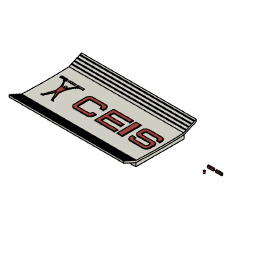
Pen_holder_ceis v9 (Autodesk Fusion 360 design; units mm, degrees)
Autodesk Fusion 360 part; units mm, degrees
sketch "Schizzo3" plane through (0, 0, 0) normal (0, 0, 1) x (1, 0, 0)
  line L0 (0, 0) -> (190, 0)
  line L1 (190, 0) -> (190, 80)
  line L2 (190, 80) -> (0, 80)
  line L3 (0, 80) -> (0, 0)
  dimension "d7" = 80
  dimension "d8" = 190
  constraint horizontal L0
  constraint vertical L1
  constraint horizontal L2
  constraint vertical L3
  constraint coincident L0.start L3.end
  measures "d7" distance of L0.start L2.end
  measures "d8" distance of L1.end L2.end
extrude "Estrusione2" add sketch "Schizzo3" along normal blind 6 makes body 1
sketch "Schizzo4" plane through (190, 0, 0) normal (1, 0, 0) x (0, 1, 0)
  line L0 (0, 0) -> (80, 0)
  line L1 (80, 0) -> (80, 6)
  line L2 (80, 6) -> (0, 6)
  line L3 (0, 6) -> (0, 0)
  line L4 (0, 6) -> (0, 5)
  line L5 (40, 5) -> (40, 9)
  line L6 (-6.5555, 6.3549) -> (30, 25)
  line L7 (30, 25) -> (86.5555, 6.3549)
  arc A0 (-6.5555, 6.3549) -> (86.5555, 6.3549) centre (40, 805.5001) ccw
  constraint coincident L2.end L3.start
  constraint coincident L3 L4.end
  constraint perpendicular L2 L4
  constraint perpendicular L2 L5
  constraint coincident L5.start A0
  constraint coincident L1.end A0
  constraint coincident L2.end A0
extrude "Estrusione3" cut sketch "Schizzo4" against normal through all contours L2 L5 A0 | L2 L6 L7 A0 | L2 L5 A0 bodies 1
sketch "Schizzo5" plane through (190, 0, 0) normal (1, 0, 0) x (0, 1, 0)
  line L0 (80, 0) -> (80, 6)
  line L1 (0, 0) -> (-20, 0)
  line L2 (-20, 0) -> (-20, 15)
  line L3 (80, 0) -> (100, 0)
  line L4 (100, 0) -> (100, 15)
  line L5 (-20, 15) -> (0, 6)
  line L6 (100, 15) -> (80, 6)
  spline S0 degree 5 poles (0, 6) (1.6, 5.9242) (4.8, 5.7791) (9.6, 5.5813) (16, 5.3581) (24, 5.1509) (32, 5.0221) (40, 4.978) (48, 5.0221) (56, 5.1509) (64, 5.3581) (70.4, 5.5813) (75.2, 5.7791) (78.4, 5.9242) (80, 6) knots 0 0 0 0 0 0 0.1 0.2 0.3 0.4 0.5 0.6 0.7 0.8 0.9 1 1 1 1 1 1
  line L7 (-20, 15) -> (-20, 18.2898)
  line L8 (100, 15) -> (100, 18.2898)
  line L9 (-18.7689, 17.7358) -> (0.7109, 8.9698)
  spline S1 degree 3 poles (0.7109, 8.9698) (18.3427, 8.1444) (35.9568, 7.8068) (53.5771, 8.1239) (62.1442, 8.2781) (70.7163, 8.5685) (79.2891, 8.9698) knots 0.007133 0.007133 0.007133 0.007133 0.670389 0.670389 0.670389 0.992867 0.992867 0.992867 0.992867
  line L10 (98.7689, 17.7358) -> (79.2891, 8.9698)
  line L11 (98.7689, 17.7358) -> (100, 18.2898)
  line L12 (-18.7689, 17.7358) -> (-20, 18.2898)
  line L13 (0.7109, 8.9698) -> (-2.9367, 10.6113)
  line L14 (-2.9367, 10.6113) -> (-2.7316, 11.0673)
  line L15 (-2.7316, 11.0673) -> (-3.6435, 11.4776)
  line L16 (-3.6435, 11.4776) -> (-3.8487, 11.0217)
  line L17 (-3.8487, 11.0217) -> (-7.4964, 12.6631)
  line L18 (-7.4964, 12.6631) -> (-7.2912, 13.1191)
  line L19 (-7.2912, 13.1191) -> (-8.2031, 13.5294)
  line L20 (-8.2031, 13.5294) -> (-8.4083, 13.0735)
  line L21 (-8.4083, 13.0735) -> (-12.056, 14.7149)
  line L22 (-12.056, 14.7149) -> (-11.8508, 15.1709)
  line L23 (-11.8508, 15.1709) -> (-12.7627, 15.5813)
  line L24 (-12.7627, 15.5813) -> (-12.9679, 15.1253)
  line L25 (-12.9679, 15.1253) -> (-16.6156, 16.7668)
  line L26 (-16.6156, 16.7668) -> (-16.4104, 17.2227)
  line L27 (-16.4104, 17.2227) -> (-17.3223, 17.6331)
  line L28 (-17.3223, 17.6331) -> (-17.5275, 17.1771)
  line L29 (0, 0) -> (40, 0)
  line L30 (40, 0) -> (40, -6)
  line L31 (82.9368, 10.6113) -> (82.7316, 11.0673)
  line L32 (82.7316, 11.0673) -> (83.6435, 11.4776)
  line L33 (83.6435, 11.4776) -> (83.8487, 11.0217)
  line L34 (87.2912, 13.1191) -> (88.2031, 13.5294)
  line L35 (87.4964, 12.6631) -> (87.2912, 13.1191)
  line L36 (88.2031, 13.5294) -> (88.4083, 13.0735)
  line L37 (92.056, 14.7149) -> (91.8508, 15.1709)
  line L38 (91.8508, 15.1709) -> (92.7627, 15.5813)
  line L39 (92.7627, 15.5813) -> (92.9679, 15.1253)
  line L40 (96.6156, 16.7668) -> (96.4104, 17.2227)
  line L41 (96.4104, 17.2227) -> (97.3223, 17.6331)
  line L42 (97.3223, 17.6331) -> (97.5275, 17.1771)
  point P0 (40, 5)
  dimension "d18" = 20
  dimension "d19" = 15
  dimension "d20" = 20
  dimension "d22" = 15
  dimension "d37" = 3
  dimension "d38" = 4
  dimension "d39" = 0.5
  dimension "d40" = 1
  dimension "d41" = 0.5
  dimension "d42" = 4
  dimension "d43" = 0.5
  dimension "d44" = 1
  dimension "d45" = 0.5
  dimension "d46" = 4
  dimension "d47" = 0.5
  dimension "d48" = 1
  dimension "d49" = 0.5
  dimension "d50" = 4
  dimension "d51" = 0.5
  dimension "d52" = 1
  dimension "d53" = 0.5
  constraint coincident L1.start L29.start
  constraint horizontal L1
  constraint perpendicular L1 L2
  constraint coincident L0.start L3.start
  constraint perpendicular L0 L3
  constraint perpendicular L3 L4
  constraint coincident L0.end L6.end
  constraint parallel L2 L7
  constraint parallel L4 L8
  constraint parallel L10 L11
  constraint parallel L9 L12
  constraint parallel L9 L13
  constraint perpendicular L9 L14
  constraint perpendicular L14 L15
  constraint perpendicular L15 L16
  constraint perpendicular L16 L17
  constraint perpendicular L17 L18
  constraint perpendicular L18 L19
  constraint perpendicular L19 L20
  constraint perpendicular L20 L21
  constraint perpendicular L9 L22
  constraint perpendicular L22 L23
  constraint perpendicular L23 L24
  constraint perpendicular L24 L25
  constraint perpendicular L9 L26
  constraint perpendicular L26 L27
  constraint perpendicular L27 L28
  constraint parallel L1 L29
  constraint perpendicular L29 L30
  constraint symmetric L13.end L30 L31.start
  constraint symmetric L14.end L30 L31.end
  constraint symmetric L15.end L30 L32.end
  constraint symmetric L16.end L30 L33.end
  constraint symmetric L17.end L30 L35.start
  constraint symmetric L18.end L30 L34.start
  constraint symmetric L19.end L30 L34.end
  constraint symmetric L20.end L30 L36.end
  constraint symmetric L21.end L30 L37.start
  constraint symmetric L22.end L30 L37.end
  constraint symmetric L23.end L30 L38.end
  constraint symmetric L24.end L30 L39.end
  constraint symmetric L25.end L30 L40.start
  constraint symmetric L26.end L30 L40.end
  constraint symmetric L27.end L30 L41.end
  constraint symmetric L28.end L30 L42.end
  measures "d18" distance of L1.start L1.end
  measures "d19" distance of L1.end L2.end
  measures "d20" distance of L0.start L3.end
  measures "d22" distance of L3.end L4.end
  measures "d38" distance of L9.end L13.end
  measures "d39" distance of L13.end L14.end
  measures "d40" distance of L14.end L15.end
  measures "d41" distance of L15.end L16.end
  measures "d42" distance of L16.end L17.end
  measures "d43" distance of L17.end L18.end
  measures "d44" distance of L18.end L19.end
  measures "d45" distance of L19.end L20.end
  measures "d46" distance of L20.end L21.end
  measures "d47" distance of L21.end L22.end
  measures "d48" distance of L22.end L23.end
  measures "d49" distance of L23.end L24.end
  measures "d50" distance of L24.end L25.end
  measures "d51" distance of L25.end L26.end
  measures "d52" distance of L26.end L27.end
  measures "d53" distance of L27.end L28.end
extrude "Estrusione5" add sketch "Schizzo5" against normal blind 190 separate body contours L5 L6 S0 L7 L8 L9 S1 L10 L11 L12 L13 L17 L21 L25 | L10 L40 L41 L42 | L9 L26 L27 L28 | L10 L37 L38 L39 | L9 L22 L23 L24 | L10 L34 L35 L36 | L9 L18 L19 L20 | L10 L31 L32 L33 | L9 L14 L15 L16 makes body 2
ref_plane "Piano di lavoro1" through (0, 0, 10) normal (0, 0, 1) x (1, 0, 0)
sketch "Schizzo8" plane through (0, 0, 10) normal (0, 0, 1) x (1, 0, 0)
  arc A0 (63.5, 56) -> (57.5, 50) centre (63.5, 50) ccw
  arc A1 (84.5, 48.2) -> (82.7, 50) centre (82.7, 48.2) ccw
  arc A2 (63.5, 32) -> (65.3, 30.2) centre (65.3, 32) ccw
  arc A3 (84.5, 24.2) -> (90.5, 30.2) centre (84.5, 30.2) ccw
  line L0 (63.5, 24.2) -> (84.5, 24.2)
  line L1 (63.5, 30.2) -> (65.3, 30.2)
  arc A4 (65.3, 50) -> (63.5, 48.2) centre (65.3, 48.2) ccw
  line L2 (57.5, 50) -> (90.5, 50)
  line L3 (57.5, 50) -> (57.5, 30.2)
  line L4 (57.5, 30.2) -> (90.5, 30.2)
  line L5 (84.5, 56) -> (63.5, 56)
  arc A5 (90.5, 50) -> (84.5, 56) centre (84.5, 50) ccw
  arc A6 (82.7, 30.2) -> (84.5, 32) centre (82.7, 32) ccw
  arc A7 (57.5, 30.2) -> (63.5, 24.2) centre (63.5, 30.2) ccw
  line L6 (84.5, 32) -> (82.7, 32)
  line L7 (84.5, 45.8) -> (90.5, 45.8)
  line L8 (63.5, 56) -> (63.5, 24.2)
  line L9 (84.5, 34.4) -> (90.5, 34.4)
  line L10 (103.5, 24.2) -> (103.5, 56)
  line L11 (97.5, 50) -> (130.5006, 50)
  line L12 (97.5, 43.1) -> (127.823, 43.1)
  line L13 (97.5, 40.1) -> (127.823, 40.1)
  line L14 (97.5, 37.1) -> (127.823, 37.1)
  line L15 (97.5, 24.2) -> (97.5, 56)
  line L16 (97.5, 24.2) -> (97.5, 49.1)
  line L17 (97.5, 56) -> (97.5, 40.1)
  line L18 (97.5, 30.2) -> (130.5, 30.2)
  line L19 (97.5, 24.2) -> (130.5, 24.2)
  line L20 (130.5, 24.2) -> (97.5, 24.2)
  line L21 (127.823, 37.1) -> (127.823, 43.1)
  line L22 (97.5, 56) -> (130.5, 56)
  line L23 (134.5, 41.008) -> (134.5, 24.2)
  line L24 (134.5, 39.175) -> (134.5, 55.9829)
  line L25 (143.5, 24.2) -> (143.5, 40.0915)
  line L26 (143.5, 40.0915) -> (143.5, 55.9829)
  arc A8 (177.5, 35.3) -> (175.7, 37.1) centre (175.7, 35.3) ccw
  line L27 (156.5, 37.1) -> (177.5, 37.1)
  line L28 (177.5, 43.1) -> (156.5, 43.1)
  line L29 (150.5, 50) -> (183.5, 50)
  arc A9 (156.5, 55.9397) -> (150.5603, 50) centre (156.5, 50) ccw
  line L30 (177.5, 56) -> (155.5, 56)
  arc A10 (183.5, 49.999) -> (177.5, 56) centre (177.5, 50) ccw
  arc A11 (183.5, 37.0982) -> (177.5, 43.1) centre (177.5, 37.1) ccw
  arc A12 (177.5, 48.2) -> (175.7, 50) centre (175.7, 48.2) ccw
  line L31 (177.5, 46.4) -> (183.5, 46.4)
  arc A13 (156.5, 44.9) -> (158.3, 43.1) centre (158.3, 44.9) ccw
  arc A14 (150.5, 43.1015) -> (156.5, 37.1) centre (156.5, 43.1) ccw
  line L32 (150.5, 30.2) -> (183.5, 30.2)
  line L33 (155.5, 24.2) -> (177.5, 24.2)
  arc A15 (150.5, 30.2) -> (156.5, 24.2) centre (156.5, 30.2) ccw
  arc A16 (156.5, 32) -> (158.3, 30.2) centre (158.3, 32) ccw
  line L34 (150.5, 33.8) -> (156.5, 33.8)
  arc A17 (177.5, 24.2) -> (183.5, 30.201) centre (177.5, 30.2) ccw
  line L35 (134.5, 55.9829) -> (143.5, 55.9829)
  line L36 (134.5, 24.2) -> (143.5, 24.2)
  line L37 (130.5, 56) -> (130.5006, 50)
  line L38 (130.5, 30.2) -> (130.5, 24.2)
  line L39 (84.5, 56) -> (84.5, 45.8)
  line L40 (84.5, 34.4) -> (84.5, 24.2)
  line L41 (90.5, 30.2) -> (90.5, 34.4)
  line L42 (90.5, 45.8) -> (90.5, 50)
  line L43 (150.5, 50) -> (150.5, 43.0985)
  line L44 (150.5, 33.8) -> (150.5, 30.2)
  line L45 (156.5, 56) -> (156.5, 37.1)
  line L46 (156.5, 33.8) -> (156.5, 24.2)
  line L47 (177.5, 24.2) -> (177.5, 43.1)
  line L48 (177.5, 46.4) -> (177.5, 56)
  line L49 (183.5, 30.199) -> (183.5, 37.1018)
  line L50 (183.5, 46.4) -> (183.5, 50.001)
  line L51 (6.5, 60.5) -> (17.5, 60.5)
  line L52 (17.5, 60.5) -> (17.5, 57.5)
  line L53 (17.5, 57.5) -> (6.5, 57.5)
  line L54 (6.5, 57.5) -> (6.5, 60.5)
  circle A18 centre (25.5, 48) radius 2
  line L55 (25.5, 48) -> (25.5, 66.722)
  line L56 (20, 57.5) -> (25.5, 57.5)
  line L57 (25.5, 57.5) -> (25.5, 60.5)
  line L58 (25.5, 60.5) -> (20, 60.5)
  line L59 (20, 60.5) -> (20, 57.5)
  line L60 (3, 16.5) -> (25.5, 16.5)
  line L61 (25.5, 16.5) -> (25.5, 62.5012)
  line L62 (25.5, 62.5012) -> (3, 62.5012)
  line L63 (3, 62.5012) -> (3, 16.5)
  line L64 (13.5, 56.5) -> (16.5, 56.5)
  line L65 (16.5, 56.5) -> (17, 55)
  line L66 (17, 55) -> (22.5, 46)
  line L67 (22.5, 46) -> (25.5, 45)
  line L68 (13.5, 56.5) -> (16, 54.5)
  line L69 (16, 54.5) -> (21, 44.5)
  line L70 (21, 44.5) -> (22.5, 34.5)
  line L71 (22.5, 34.5) -> (17.5, 19.5)
  line L72 (17.5, 19.5) -> (15, 17.5)
  line L73 (15, 17.5) -> (18.5, 17.5)
  line L74 (18.5, 17.5) -> (25.5, 32.5)
  line L75 (25.5, 60.5) -> (31, 60.5)
  line L76 (31, 60.5) -> (31, 57.5)
  line L77 (31, 57.5) -> (25.5, 57.5)
  line L78 (33.5, 60.5) -> (33.5, 57.5)
  line L79 (44.5, 60.5) -> (33.5, 60.5)
  line L80 (44.5, 57.5) -> (44.5, 60.5)
  line L81 (33.5, 57.5) -> (44.5, 57.5)
  line L82 (37.5, 56.5) -> (34.5, 56.5)
  line L83 (34.5, 56.5) -> (34, 55)
  line L84 (34, 55) -> (28.5, 46)
  line L85 (37.5, 56.5) -> (35, 54.5)
  line L86 (35, 54.5) -> (30, 44.5)
  circle A19 centre (25.5, 48) radius 2
  line L87 (28.5, 46) -> (25.5, 45)
  line L88 (30, 44.5) -> (28.5, 34.5)
  line L89 (28.5, 34.5) -> (33.5, 19.5)
  line L90 (32.5, 17.5) -> (25.5, 32.5)
  line L91 (36, 17.5) -> (32.5, 17.5)
  line L92 (33.5, 19.5) -> (36, 17.5)
  line L93 (25.5, 62.5012) -> (48, 62.5012)
  line L94 (48, 62.5012) -> (48, 16.5)
  line L95 (48, 16.5) -> (25.5, 16.5)
  point P0 (143.5, 55.9829)
  point P1 (158.3, 48.2)
  point P2 (177.5, 37.1)
  point P3 (156.5, 48.2)
  point P4 (158.3, 50)
  point P5 (117.5, -48.5)
  point P6 (150.6297, 56)
  constraint horizontal L0
  constraint vertical L41
  constraint horizontal L5
  constraint vertical L3
  constraint perpendicular L0 L8
  constraint perpendicular L5 L39
  constraint perpendicular L2 L41
  constraint perpendicular L4 L41
  constraint coincident A0.centre L8
  constraint coincident A0.centre L2
  constraint coincident A5.centre L2
  constraint coincident A5.centre L39
  constraint coincident L1.start L8
  constraint coincident L1.start L4
  constraint coincident A3.centre L4
  constraint coincident A3.centre L39
  constraint coincident L1.start A7.centre
  constraint perpendicular L1 L8
  constraint tangent A2 L8
  constraint coincident A6.end L39
  constraint perpendicular L6 L39
  constraint coincident A6.centre L6.end
  constraint tangent A1 L2
  constraint coincident A4.end L8
  constraint coincident A4.start L2
  constraint coincident A2.start L8
  constraint coincident A6.start L4
  constraint coincident A1.end L2
  constraint coincident A1.start L39
  constraint coincident L7.end L41
  constraint perpendicular L7 L41
  constraint coincident L9.start L39
  constraint perpendicular L9 L41
  constraint perpendicular L16 L19
  constraint horizontal L20
  constraint coincident L10.start L19
  constraint horizontal L11
  constraint coincident L11.start L15
  constraint coincident L11.start L17
  constraint coincident L18.start L16
  constraint coincident L18.start L15
  constraint coincident L14.start L15
  constraint coincident L13.start L15
  constraint parallel L12 L13
  constraint coincident P0 L26.end
  constraint horizontal L33
  constraint vertical L49
  constraint horizontal L30
  constraint vertical L43
  constraint coincident L29.end L49
  constraint perpendicular L29 L49
  constraint coincident L32.end L49
  constraint perpendicular L32 L49
  constraint coincident P6 L30
  constraint coincident L45.start L30
  constraint perpendicular L32 L45
  constraint perpendicular L30 L47
  constraint coincident A9.centre L45
  constraint coincident A9.centre L29
  constraint coincident A17.centre L47
  constraint coincident A17.centre L32
  constraint coincident A10.centre L47
  constraint coincident A10.centre L29
  constraint coincident L34.start L43
  constraint coincident L34.end L45
  constraint perpendicular L34 L45
  constraint coincident L31.start L47
  constraint coincident L31.end L49
  constraint coincident A9.start L45
  constraint coincident A9.end L29
  constraint coincident A17.end L49
  constraint coincident A10.start L49
  constraint tangent L29 A12
  constraint coincident P3 L45
  constraint coincident P4 L29
  constraint coincident A12.end L29
  constraint coincident A12.start L47
  constraint coincident A16.end L32
  constraint coincident A16.start L45
  constraint perpendicular L28 L47
  constraint coincident L28.end L45
  constraint coincident P2 L47
  constraint perpendicular L27 L47
  constraint tangent A8 L27
  constraint coincident L28.end A14.centre
  constraint coincident P2 L27.end
  constraint coincident A14.start L43
  constraint coincident A11.start L49
  constraint coincident A8.end L27
  constraint coincident A8.start L47
  constraint coincident A13.end L28
  constraint coincident A13.start L45
  constraint perpendicular L26 L35
  constraint perpendicular L25 L36
  constraint perpendicular L20 L38
  constraint coincident L21 L13.end
  constraint collinear L39 L40
  constraint collinear L41 L42
  constraint coincident A17 L49.start
  constraint coincident A10 L50.end
  constraint coincident A14 L43.end
  constraint collinear L43 L44
  constraint collinear L45 L46
  constraint collinear L47 L48
  constraint coincident A11 L49.end
  constraint collinear L49 L50
  constraint horizontal L51
  constraint vertical L52
  constraint horizontal L53
  constraint vertical L54
  constraint coincident A18.centre L55.start
  constraint horizontal L56
  constraint vertical L57
  constraint horizontal L58
  constraint vertical L59
  constraint coincident L55 L57.end
  constraint horizontal L60
  constraint vertical L61
  constraint horizontal L62
  constraint vertical L63
  constraint coincident L55 L61.end
  constraint parallel L53 L64
  constraint coincident L61 L67.end
  constraint horizontal L73
  constraint coincident L61 L74.end
  constraint symmetric L51.start L61 L79.start
  constraint symmetric L51.end L61 L78.start
  constraint symmetric L52.end L61 L78.end
  constraint symmetric L53.end L61 L80.start
  constraint symmetric A18 L61 A19
  constraint symmetric L56.start L61 L76.end
  constraint symmetric L56.end L61 L57.start
  constraint symmetric L57.end L61 L58.start
  constraint symmetric L58.end L61 L75.end
  constraint symmetric L61 L64.start L82.start
  constraint symmetric L61 L64.end L82.end
  constraint symmetric L61 L65.end L83.end
  constraint symmetric L61 L66.end L84.end
  constraint symmetric L61 L67.end L87.end
  constraint symmetric L61 L68.end L85.end
  constraint symmetric L61 L69.end L86.end
  constraint symmetric L61 L70.end L88.end
  constraint symmetric L61 L71.end L89.end
  constraint symmetric L61 L72.end L91.start
  constraint symmetric L61 L73.end L90.start
  constraint symmetric L61 L74.end L90.end
  constraint symmetric L55 L60.start L94.end
  constraint symmetric L55 L60.end L61.start
  constraint symmetric L55 L61.end L62.start
  constraint symmetric L55 L62.end L93.end
extrude "Estrusione6" cut sketch "Schizzo8" against normal blind 4 contours A0 L2 L8 | L2 L5 L8 L39 | L2 L3 L4 L8 | L2 A5 L39 | A4 L2 L8 | L4 A7 L8 | L2 L7 L39 L42 | A1 L2 L39 | A2 L1 L4 L8 | L0 L1 L4 L8 L40 | A3 L4 L40 | L4 A6 L40 | L4 L9 L40 L41 | L10 L15 L16 L18 L19 L20 | L10 L18 L19 L20 L38 | L10 L14 L15 L16 L18 | L10 L13 L14 L15 L16 | L10 L13 L14 L21 | L10 L12 L13 L15 L16 L17 | L10 L12 L13 L21 | L10 L11 L12 L15 L16 L17 | L10 L11 L15 L17 L22 | L10 L11 L22 L37 | L23 L24 L25 L26 L35 L36 | A8 L27 L47 | A11 L32 L47 L49 | L27 L28 L45 L47 | L32 L33 L46 L47 | L32 A17 L47 | L29 A14 L43 L45 | L32 A16 L46 | L28 A13 L45 | L32 A15 L46 | L32 L34 L44 L46 | L29 L30 L45 L48 | L29 A9 L45 | L29 A12 L48 | L29 A10 L48 | L29 L31 L48 L50 | L51 L52 L53 L54 | A18 L55 L61 A19 | A18 L55 L61 A19 | L55 L56 L57 L58 L59 L61 | L55 L57 L61 L75 L76 L77 | L61 L82 L83 L84 L85 L86 L87 L88 L89 L90 L91 L92 | L61 L64 L65 L66 L67 L68 L69 L70 L71 L72 L73 L74 | L78 L79 L80 L81 bodies 2
sketch "Schizzo9" plane through (0, 0, 0) normal (0, 0, 1) x (1, 0, 0)
  line L0 (243.5, 56.5) -> (246, 54.5)
  line L1 (266, 17.5) -> (262.5, 17.5)
  line L2 (246, 54.5) -> (251, 44.5)
  line L3 (252.5, 46) -> (255.5, 45)
  line L4 (245, 17.5) -> (248.5, 17.5)
  line L5 (247, 55) -> (252.5, 46)
  line L6 (263.5, 19.5) -> (266, 17.5)
  line L7 (248.5, 17.5) -> (255.5, 32.5)
  line L8 (252.5, 34.5) -> (247.5, 19.5)
  line L9 (243.5, 56.5) -> (246.5, 56.5)
  line L10 (258.5, 34.5) -> (263.5, 19.5)
  line L11 (247.5, 19.5) -> (245, 17.5)
  line L12 (260, 44.5) -> (258.5, 34.5)
  line L13 (251, 44.5) -> (252.5, 34.5)
  line L14 (262.5, 17.5) -> (255.5, 32.5)
  line L15 (264, 55) -> (258.5, 46)
  line L16 (267.5, 56.5) -> (264.5, 56.5)
  line L17 (267.5, 56.5) -> (265, 54.5)
  line L18 (265, 54.5) -> (260, 44.5)
  line L19 (264.5, 56.5) -> (264, 55)
  line L20 (246.5, 56.5) -> (247, 55)
  line L21 (258.5, 46) -> (255.5, 45)
  arc A0 (391, 43.1014) -> (396.5, 37.6) centre (396.5, 43.1) ccw
  line L22 (396.5, 37.6) -> (415.7, 37.6)
  arc A1 (418, 35.3) -> (415.7, 37.6) centre (415.7, 35.3) ccw
  line L23 (418, 32) -> (418, 35.3)
  arc A2 (415.7, 29.7) -> (418, 32) centre (415.7, 32) ccw
  line L24 (398.3, 29.7) -> (415.7, 29.7)
  arc A3 (396, 32) -> (398.3, 29.7) centre (398.3, 32) ccw
  line L25 (396, 33.3) -> (396, 32)
  line L26 (391, 33.3) -> (396, 33.3)
  line L27 (391, 33.3) -> (391, 30.2)
  arc A4 (391, 30.2) -> (396.5, 24.7) centre (396.5, 30.2) ccw
  line L28 (423, 30.199) -> (423, 37.1018)
  line L29 (396.5, 24.7) -> (417.5, 24.7)
  arc A5 (417.5, 24.7) -> (423, 30.201) centre (417.5, 30.2) ccw
  arc A6 (423, 37.0983) -> (417.5, 42.6) centre (417.5, 37.1) ccw
  line L30 (417.5, 42.6) -> (398.3, 42.6)
  arc A7 (396, 44.9) -> (398.3, 42.6) centre (398.3, 44.9) ccw
  line L31 (396, 48.2) -> (396, 44.9)
  arc A8 (398.3, 50.5) -> (396, 48.2) centre (398.3, 48.2) ccw
  line L32 (398.3, 50.5) -> (415.7, 50.5)
  arc A9 (418, 48.2) -> (415.7, 50.5) centre (415.7, 48.2) ccw
  line L33 (418, 46.9) -> (418, 48.2)
  line L34 (418, 46.9) -> (423, 46.9)
  line L35 (423, 46.9) -> (423, 50.001)
  arc A10 (423, 49.9991) -> (417.5, 55.5) centre (417.5, 50) ccw
  line L36 (417.5, 55.5) -> (396.5, 55.5)
  arc A11 (396.5, 55.5) -> (391, 50) centre (396.5, 50) ccw
  line L37 (391, 50) -> (391, 43.0985)
  line L38 (375, 39.175) -> (375, 41.008)
  line L39 (375, 41.008) -> (375, 55.4829)
  line L40 (375, 55.4829) -> (383, 55.4829)
  line L41 (383, 40.0915) -> (383, 55.4829)
  line L42 (383, 24.7) -> (383, 40.0915)
  line L43 (375, 24.7) -> (383, 24.7)
  line L44 (375, 39.175) -> (375, 24.7)
  line L45 (298, 50) -> (298, 30.2)
  arc A12 (298, 30.2) -> (303.5, 24.7) centre (303.5, 30.2) ccw
  line L46 (303.5, 24.7) -> (324.5, 24.7)
  arc A13 (324.5, 24.7) -> (330, 30.2) centre (324.5, 30.2) ccw
  line L47 (330, 30.2) -> (330, 33.9)
  line L48 (325, 33.9) -> (330, 33.9)
  line L49 (325, 33.9) -> (325, 32)
  arc A14 (322.7, 29.7) -> (325, 32) centre (322.7, 32) ccw
  line L50 (305.3, 29.7) -> (322.7, 29.7)
  arc A15 (303, 32) -> (305.3, 29.7) centre (305.3, 32) ccw
  line L51 (303, 48.2) -> (303, 32)
  arc A16 (305.3, 50.5) -> (303, 48.2) centre (305.3, 48.2) ccw
  line L52 (305.3, 50.5) -> (322.7, 50.5)
  arc A17 (325, 48.2) -> (322.7, 50.5) centre (322.7, 48.2) ccw
  line L53 (325, 48.2) -> (325, 46.3)
  line L54 (325, 46.3) -> (330, 46.3)
  line L55 (330, 46.3) -> (330, 50)
  arc A18 (330, 50) -> (324.5, 55.5) centre (324.5, 50) ccw
  line L56 (324.5, 55.5) -> (303.5, 55.5)
  arc A19 (303.5, 55.5) -> (298, 50) centre (303.5, 50) ccw
  line L57 (338, 40.1) -> (338, 49.1)
  line L58 (338, 24.7) -> (338, 40.1)
  line L59 (338, 24.7) -> (370, 24.7)
  line L60 (370, 29.7) -> (370, 24.7)
  line L61 (343, 29.7) -> (370, 29.7)
  line L62 (343, 29.7) -> (343, 37.6)
  line L63 (343, 37.6) -> (367.323, 37.6)
  line L64 (367.323, 37.6) -> (367.323, 42.6)
  line L65 (343, 42.6) -> (367.323, 42.6)
  line L66 (343, 42.6) -> (343, 50.5)
  line L67 (343, 50.5) -> (370.0006, 50.5)
  line L68 (370.0001, 55.5) -> (370.0006, 50.5)
  line L69 (338, 55.5) -> (370.0001, 55.5)
  line L70 (338, 55.5) -> (338, 49.1)
  circle A20 centre (255.5, 48) radius 1.5
  line L71 (250.5, 58) -> (255.5, 58)
  line L72 (260.5, 58) -> (255.5, 58)
  line L73 (260.5, 60) -> (260.5, 58)
  line L74 (255.5, 60) -> (260.5, 60)
  line L75 (255.5, 60) -> (250.5, 60)
  line L76 (250.5, 60) -> (250.5, 58)
  line L77 (264, 58) -> (274, 58)
  line L78 (274, 58) -> (274, 60)
  line L79 (274, 60) -> (264, 60)
  line L80 (264, 60) -> (264, 58)
  line L81 (247, 58) -> (237, 58)
  line L82 (237, 58) -> (237, 60)
  line L83 (237, 60) -> (247, 60)
  line L84 (247, 60) -> (247, 58)
  line L85 (252.3343, 45.7917) -> (255.5, 44.7365)
  line L86 (258.6657, 45.7917) -> (255.5, 44.7365)
  line L87 (264.2282, 54.8939) -> (258.6657, 45.7917)
  line L88 (264.6802, 56.25) -> (264.2282, 54.8939)
  line L89 (266.7873, 56.25) -> (264.6802, 56.25)
  line L90 (266.7873, 56.25) -> (264.8009, 54.6609)
  line L91 (264.8009, 54.6609) -> (259.7587, 44.5763)
  line L92 (259.7587, 44.5763) -> (258.2439, 34.4778)
  line L93 (258.2439, 34.4778) -> (263.2862, 19.3509)
  line L94 (263.2862, 19.3509) -> (265.2873, 17.75)
  line L95 (265.2873, 17.75) -> (262.6592, 17.75)
  line L96 (262.6592, 17.75) -> (255.5, 33.0912)
  line L97 (248.3408, 17.75) -> (255.5, 33.0912)
  line L98 (245.7127, 17.75) -> (248.3408, 17.75)
  line L99 (247.7138, 19.3509) -> (245.7127, 17.75)
  line L100 (252.7561, 34.4778) -> (247.7138, 19.3509)
  line L101 (251.2413, 44.5763) -> (252.7561, 34.4778)
  line L102 (246.1991, 54.6609) -> (251.2413, 44.5763)
  line L103 (244.2127, 56.25) -> (246.1991, 54.6609)
  line L104 (244.2127, 56.25) -> (246.3198, 56.25)
  line L105 (246.3198, 56.25) -> (246.7718, 54.8939)
  line L106 (246.7718, 54.8939) -> (252.3343, 45.7917)
  point P0 (390.6297, 56)
  point P1 (383.5, 55.9829)
  point P2 (398.3, 48.2)
  point P3 (417.5, 37.1)
  dimension "d82" = 0.25
  constraint horizontal L4
  constraint tangent A11 L37
  constraint tangent A10 L36
  constraint tangent L36 A11
  constraint tangent A8 L32
  constraint tangent L32 A9
  constraint tangent A6 L30
  constraint tangent L30 A7
  constraint tangent L29 A5
  constraint tangent L23 A2
  constraint tangent A0 L22
  constraint tangent L22 A1
  constraint tangent A1 L23
  constraint tangent A2 L24
  constraint tangent L24 A3
  constraint tangent A3 L25
  constraint tangent L27 A4
  constraint tangent L45 A19
  constraint tangent L49 A14
  constraint tangent L45 A12
  constraint tangent A14 L50
  constraint tangent L50 A15
  constraint tangent A16 L52
  constraint tangent L52 A17
  constraint tangent A17 L53
  constraint tangent L55 A18
  constraint tangent A18 L56
  constraint tangent L56 A19
extrude "Estrusione7" add sketch "Schizzo9" along normal blind 3 separate body contours A0 L22 A1 L23 A2 L24 A3 L25 L26 L27 A4 L28 L29 A5 A6 L30 A7 L31 A8 L32 A9 L33 L34 L35 A10 L36 A11 L37 | L38 L39 L40 L41 L42 L43 L44 | L45 A12 L46 A13 L47 L48 L49 A14 L50 A15 L51 A16 L52 A17 L53 L54 L55 A18 L56 A19 | L57 L58 L59 L60 L61 L62 L63 L64 L65 L66 L67 L68 L69 L70 makes body 3 at (339.6667, 39.2667, 0) makes body 4 at (380.3333, 34.961, 0) makes body 5 at (316.9, 53.8333, 0) makes body 6 at (409.9, 53.8333, 3)
move_body "Allinea1" bodies 5 to x (1, 0, 0) y (0, 1, 0) z (0, 0, 1) at (-240, -0.5, 6)
move_body "Allinea2" bodies 3 to x (1, 0, 0) y (0, 1, 0) z (0, 0, 1) at (-240, -0.5, 6)
move_body "Allinea3" bodies 4 to x (1, 0, 0) y (0, 1, 0) z (0, 0, 1) at (-240, -0.5, 6)
move_body "Allinea4" bodies 6 to x (1, 0, 0) y (0, 1, 0) z (0, 0, 1) at (-240, -0.5, 6)
extrude "Estrusione8" add sketch "Schizzo9" along normal blind 3 separate body contours A20 | L71 L72 L73 L74 L75 L76 | L77 L78 L79 L80 | L81 L82 L83 L84 | L85 L86 L87 L88 L89 L90 L91 L92 L93 L94 L95 L96 L97 L98 L99 L100 L101 L102 L103 L104 L105 L106 makes body 7 at (270.6667, 60, 1) makes body 8 at (257.1667, 60, 1) makes body 9 at (255.5, 37.8974, 0) makes body 10 at (243.6667, 58, 1) makes body 11 at (255.9063, 49.4439, 2)
move_body "Allinea5" bodies 9 to x (1, 0, 0) y (0, 1, 0) z (0, 0, 1) at (-229.7233, -0.25, 6)
move_body "Allinea6" bodies 10 to x (1, 0, 0) y (0, 1, 0) z (0, 0, 1) at (-230, 0.5, 5.6388)
